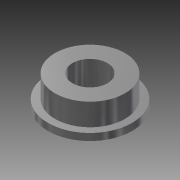
# Autodesk Inventor part: Bearing_SMF63ZZ
Saved by Autodesk Inventor 2015 (Build 190159000, 159)
## iProperties
Created: 2015-05-23
Part Number: Bearing_SMF63ZZ
Material: ステンレス鋼
Document SubType Name: Modeling
Designer: kenta
Density: 8 g/cm^3
Appearance: 半つや出し
Mass: 0.48383 g
Surface Area: 1.40241 cm^2
Volume: 0.0604788 cm^3
Author: kenta
Autodesk Inventor part; units mm, degrees
ref_plane "YZ Plane" through (0, 0, 0) normal (1, 0, 0) x (0, 1, 0)
ref_plane "XZ Plane" through (0, 0, 0) normal (0, 1, 0) x (-1, 0, 0)
ref_plane "XY Plane" through (0, 0, 0) normal (0, 0, 1) x (1, 0, 0)
sketch "スケッチ1" plane through (0, 0, 0) normal (0, 0, 1) x (1, 0, 0)
  circle A0 centre (0, 0) radius 3.6
  dimension "d0" = 7.2
  constraints: 1 centre point, 1 coincident
  measures "d0" diameter of A0
extrude "押し出し1" add sketch "スケッチ1" along normal blind 0.6
sketch "スケッチ2" plane through (0, 0, 0.6) normal (0, 0, 1) x (1, 0, 0)
  circle A0 centre (0, 0) radius 3
  dimension "d3" = 6
  constraints: 1 centre point, 1 coincident
  measures "d3" diameter of A0
extrude "押し出し2" add sketch "スケッチ2" along normal blind 1.9
sketch "スケッチ3" plane through (0, 0, 2.5) normal (0, 0, 1) x (1, 0, 0)
  circle A0 centre (0, 0) radius 1.5
  dimension "d6" = 3
  constraints: 1 centre point, 1 coincident
  measures "d6" diameter of A0
extrude "押し出し3" cut sketch "スケッチ3" against normal blind 5
